Autodesk Inventor part; units mm, degrees
(part 2 of 2)
sketch "Sketch3" plane through (-0.0003, -144.9621, -142.4319) normal (0, 0, -1) x (-1, 0, 0)
  line L0 (-10.1604, 66.049) -> (-10.1604, 136.1421) construction
  line L1 (-10.1604, 136.1421) -> (-1.0068, 136.1421) construction
  line L2 (-1.0068, 136.1421) -> (-1.0068, 66.049) construction
  line L3 (-1.0068, 66.049) -> (-10.1604, 66.049) construction
  spline S0 degree 2 poles (-7.5802, 71.9161) (-7.0615, 71.9161) (-6.128, 71.5465) (-5.8038, 71.2159) knots 0 0 0 1 2 2 2
  spline S1 degree 2 poles (-5.8038, 71.2159) (-5.3954, 70.801) (-4.974, 69.6794) (-4.974, 68.8237) knots 0 0 0 1 2 2 2
  line L4 (-4.974, 68.8237) -> (-4.974, 67.9225)
  line L5 (-4.974, 67.9225) -> (-1.9918, 67.9225)
  line L6 (-1.9918, 67.9225) -> (-1.9918, 66.8593)
  line L7 (-1.9918, 66.8593) -> (-9.9918, 66.8593)
  line L8 (-9.9918, 66.8593) -> (-9.9918, 68.8691)
  spline S2 degree 2 poles (-9.9918, 68.8691) (-9.9918, 69.5822) (-9.7585, 70.5806) (-9.4927, 70.9631) knots 0 0 0 1 2 2 2
  spline S3 degree 2 poles (-9.4927, 70.9631) (-9.188, 71.4104) (-8.2479, 71.9161) (-7.5802, 71.9161) knots 0 0 0 1 2 2 2
  spline S4 degree 2 poles (-7.5478, 70.8075) (-7.9627, 70.8075) (-8.5721, 70.5222) (-8.7666, 70.2305) knots 0 0 0 1 2 2 2
  spline S5 degree 2 poles (-8.7666, 70.2305) (-8.9351, 69.9777) (-9.0713, 69.3034) (-9.0713, 68.8042) knots 0 0 0 1 2 2 2
  line L9 (-9.0713, 68.8042) -> (-9.0713, 67.9225)
  line L10 (-9.0713, 67.9225) -> (-5.8816, 67.9225)
  line L11 (-5.8816, 67.9225) -> (-5.8816, 68.6486)
  spline S6 degree 2 poles (-5.8816, 68.6486) (-5.8816, 69.2969) (-6.0891, 70.0943) (-6.3614, 70.3537) knots 0 0 0 1 2 2 2
  spline S7 degree 2 poles (-6.3614, 70.3537) (-6.6012, 70.5935) (-7.1653, 70.8075) (-7.5478, 70.8075) knots 0 0 0 1 2 2 2
  line L12 (-1.9918, 79.1187) -> (-1.9918, 77.7378)
  line L13 (-1.9918, 77.7378) -> (-5.175, 75.2094)
  line L14 (-5.175, 75.2094) -> (-5.175, 73.9906)
  line L15 (-5.175, 73.9906) -> (-1.9918, 73.9906)
  line L16 (-1.9918, 73.9906) -> (-1.9918, 72.9274)
  line L17 (-1.9918, 72.9274) -> (-9.9918, 72.9274)
  line L18 (-9.9918, 72.9274) -> (-9.9918, 74.989)
  spline S8 degree 2 poles (-9.9918, 74.989) (-9.9918, 75.6762) (-9.8427, 76.6033) (-9.5705, 77.0247) knots 0 0 0 1 2 2 2
  spline S9 degree 2 poles (-9.5705, 77.0247) (-9.2982, 77.446) (-8.4489, 77.9323) (-7.82, 77.9323) knots 0 0 0 1 2 2 2
  spline S10 degree 2 poles (-7.82, 77.9323) (-6.9448, 77.9323) (-5.7585, 77.0376) (-5.4732, 76.2726) knots 0 0 0 1 2 2 2
  line L19 (-5.4732, 76.2726) -> (-1.9918, 79.1187)
  spline S11 degree 2 poles (-7.7358, 76.8237) (-8.0858, 76.8237) (-8.6239, 76.5773) (-8.799, 76.318) knots 0 0 0 1 2 2 2
  spline S12 degree 2 poles (-8.799, 76.318) (-8.9481, 76.0911) (-9.0713, 75.4882) (-9.0713, 75.0473) knots 0 0 0 1 2 2 2
  line L20 (-9.0713, 75.0473) -> (-9.0713, 73.9906)
  line L21 (-9.0713, 73.9906) -> (-6.0632, 73.9906)
  line L22 (-6.0632, 73.9906) -> (-6.0632, 74.9242)
  spline S13 degree 2 poles (-6.0632, 74.9242) (-6.0632, 75.3845) (-6.2252, 76.117) (-6.4781, 76.3699) knots 0 0 0 1 2 2 2
  spline S14 degree 2 poles (-6.4781, 76.3699) (-6.6985, 76.6033) (-7.3209, 76.8237) (-7.7358, 76.8237) knots 0 0 0 1 2 2 2
  spline S15 degree 2 poles (-9.0777, 85.4136) (-8.5461, 85.8674) (-6.9902, 86.3731) (-5.9918, 86.3731) knots 0 0 0 1 2 2 2
  spline S16 degree 2 poles (-5.9918, 86.3731) (-5.0194, 86.3731) (-3.444, 85.8804) (-2.9124, 85.4136) knots 0 0 0 1 2 2 2
  spline S17 degree 2 poles (-2.9124, 85.4136) (-2.3549, 84.9209) (-1.8233, 83.6178) (-1.8233, 82.8334) knots 0 0 0 1 2 2 2
  spline S18 degree 2 poles (-1.8233, 82.8334) (-1.8233, 82.023) (-2.3743, 80.7264) (-2.9124, 80.2532) knots 0 0 0 1 2 2 2
  spline S19 degree 2 poles (-2.9124, 80.2532) (-3.444, 79.7929) (-5.0064, 79.3002) (-5.9918, 79.3002) knots 0 0 0 1 2 2 2
  spline S20 degree 2 poles (-5.9918, 79.3002) (-6.9967, 79.3002) (-8.5267, 79.7994) (-9.0777, 80.2597) knots 0 0 0 1 2 2 2
  spline S21 degree 2 poles (-9.0777, 80.2597) (-9.6094, 80.7264) (-10.1604, 82.0295) (-10.1604, 82.8334) knots 0 0 0 1 2 2 2
  spline S22 degree 2 poles (-10.1604, 82.8334) (-10.1604, 83.6503) (-9.5899, 84.9598) (-9.0777, 85.4136) knots 0 0 0 1 2 2 2
  spline S23 degree 2 poles (-5.9918, 85.2645) (-6.7828, 85.2645) (-8.0081, 84.9209) (-8.41, 84.6097) knots 0 0 0 1 2 2 2
  spline S24 degree 2 poles (-8.41, 84.6097) (-8.8249, 84.2921) (-9.2398, 83.3974) (-9.2398, 82.8399) knots 0 0 0 1 2 2 2
  spline S25 degree 2 poles (-9.2398, 82.8399) (-9.2398, 82.2629) (-8.8379, 81.3942) (-8.41, 81.0636) knots 0 0 0 1 2 2 2
  spline S26 degree 2 poles (-8.41, 81.0636) (-8.0016, 80.7459) (-6.7698, 80.4088) (-5.9918, 80.4088) knots 0 0 0 1 2 2 2
  spline S27 degree 2 poles (-5.9918, 80.4088) (-4.4165, 80.4088) (-2.7439, 81.7313) (-2.7439, 82.8399) knots 0 0 0 1 2 2 2
  spline S28 degree 2 poles (-2.7439, 82.8399) (-2.7439, 83.9485) (-4.4165, 85.2645) (-5.9918, 85.2645) knots 0 0 0 1 2 2 2
  line L23 (-1.9918, 89.4071) -> (-9.0453, 89.4071)
  line L24 (-9.0453, 89.4071) -> (-9.0453, 86.7232)
  line L25 (-9.0453, 86.7232) -> (-9.9918, 86.7232)
  line L26 (-9.9918, 86.7232) -> (-9.9918, 93.1543)
  line L27 (-9.9918, 93.1543) -> (-9.0453, 93.1543)
  line L28 (-9.0453, 93.1543) -> (-9.0453, 90.4704)
  line L29 (-9.0453, 90.4704) -> (-1.9918, 90.4704)
  line L30 (-1.9918, 90.4704) -> (-1.9918, 89.4071)
  spline S29 degree 2 poles (-9.0777, 99.6243) (-8.5461, 100.0781) (-6.9902, 100.5838) (-5.9918, 100.5838) knots 0 0 0 1 2 2 2
  spline S30 degree 2 poles (-5.9918, 100.5838) (-5.0194, 100.5838) (-3.444, 100.0911) (-2.9124, 99.6243) knots 0 0 0 1 2 2 2
  spline S31 degree 2 poles (-2.9124, 99.6243) (-2.3549, 99.1316) (-1.8233, 97.8285) (-1.8233, 97.0441) knots 0 0 0 1 2 2 2
  spline S32 degree 2 poles (-1.8233, 97.0441) (-1.8233, 96.2337) (-2.3743, 94.9371) (-2.9124, 94.4639) knots 0 0 0 1 2 2 2
  spline S33 degree 2 poles (-2.9124, 94.4639) (-3.444, 94.0036) (-5.0064, 93.5109) (-5.9918, 93.5109) knots 0 0 0 1 2 2 2
  spline S34 degree 2 poles (-5.9918, 93.5109) (-6.9967, 93.5109) (-8.5267, 94.0101) (-9.0777, 94.4704) knots 0 0 0 1 2 2 2
  spline S35 degree 2 poles (-9.0777, 94.4704) (-9.6094, 94.9371) (-10.1604, 96.2402) (-10.1604, 97.0441) knots 0 0 0 1 2 2 2
  spline S36 degree 2 poles (-10.1604, 97.0441) (-10.1604, 97.861) (-9.5899, 99.1705) (-9.0777, 99.6243) knots 0 0 0 1 2 2 2
  spline S37 degree 2 poles (-5.9918, 99.4752) (-6.7828, 99.4752) (-8.0081, 99.1316) (-8.41, 98.8204) knots 0 0 0 1 2 2 2
  spline S38 degree 2 poles (-8.41, 98.8204) (-8.8249, 98.5028) (-9.2398, 97.6081) (-9.2398, 97.0506) knots 0 0 0 1 2 2 2
  spline S39 degree 2 poles (-9.2398, 97.0506) (-9.2398, 96.4736) (-8.8379, 95.6049) (-8.41, 95.2742) knots 0 0 0 1 2 2 2
  spline S40 degree 2 poles (-8.41, 95.2742) (-8.0016, 94.9566) (-6.7698, 94.6195) (-5.9918, 94.6195) knots 0 0 0 1 2 2 2
  spline S41 degree 2 poles (-5.9918, 94.6195) (-4.4165, 94.6195) (-2.7439, 95.942) (-2.7439, 97.0506) knots 0 0 0 1 2 2 2
  spline S42 degree 2 poles (-2.7439, 97.0506) (-2.7439, 98.1592) (-4.4165, 99.4752) (-5.9918, 99.4752) knots 0 0 0 1 2 2 2
  line L31 (-1.9918, 103.6178) -> (-9.0453, 103.6178)
  line L32 (-9.0453, 103.6178) -> (-9.0453, 100.9339)
  line L33 (-9.0453, 100.9339) -> (-9.9918, 100.9339)
  line L34 (-9.9918, 100.9339) -> (-9.9918, 107.365)
  line L35 (-9.9918, 107.365) -> (-9.0453, 107.365)
  line L36 (-9.0453, 107.365) -> (-9.0453, 104.6811)
  line L37 (-9.0453, 104.6811) -> (-1.9918, 104.6811)
  line L38 (-1.9918, 104.6811) -> (-1.9918, 103.6178)
  line L39 (-9.9918, 113.7767) -> (-5.5316, 111.0733)
  line L40 (-5.5316, 111.0733) -> (-1.9918, 111.0733)
  line L41 (-1.9918, 111.0733) -> (-1.9918, 110.0101)
  line L42 (-1.9918, 110.0101) -> (-5.4213, 110.0101)
  line L43 (-5.4213, 110.0101) -> (-9.9918, 107.3067)
  line L44 (-9.9918, 107.3067) -> (-9.9918, 108.4866)
  line L45 (-9.9918, 108.4866) -> (-6.4716, 110.5482)
  line L46 (-6.4716, 110.5482) -> (-9.9918, 112.6486)
  line L47 (-9.9918, 112.6486) -> (-9.9918, 113.7767)
  spline S43 degree 2 poles (-7.5802, 119.5725) (-7.0615, 119.5725) (-6.128, 119.2029) (-5.8038, 118.8723) knots 0 0 0 1 2 2 2
  spline S44 degree 2 poles (-5.8038, 118.8723) (-5.3954, 118.4574) (-4.974, 117.3358) (-4.974, 116.4801) knots 0 0 0 1 2 2 2
  line L48 (-4.974, 116.4801) -> (-4.974, 115.5789)
  line L49 (-4.974, 115.5789) -> (-1.9918, 115.5789)
  line L50 (-1.9918, 115.5789) -> (-1.9918, 114.5157)
  line L51 (-1.9918, 114.5157) -> (-9.9918, 114.5157)
  line L52 (-9.9918, 114.5157) -> (-9.9918, 116.5255)
  spline S45 degree 2 poles (-9.9918, 116.5255) (-9.9918, 117.2386) (-9.7585, 118.237) (-9.4927, 118.6195) knots 0 0 0 1 2 2 2
  spline S46 degree 2 poles (-9.4927, 118.6195) (-9.188, 119.0668) (-8.2479, 119.5725) (-7.5802, 119.5725) knots 0 0 0 1 2 2 2
  spline S47 degree 2 poles (-7.5478, 118.4639) (-7.9627, 118.4639) (-8.5721, 118.1786) (-8.7666, 117.8869) knots 0 0 0 1 2 2 2
  spline S48 degree 2 poles (-8.7666, 117.8869) (-8.9351, 117.6341) (-9.0713, 116.9598) (-9.0713, 116.4606) knots 0 0 0 1 2 2 2
  line L53 (-9.0713, 116.4606) -> (-9.0713, 115.5789)
  line L54 (-9.0713, 115.5789) -> (-5.8816, 115.5789)
  line L55 (-5.8816, 115.5789) -> (-5.8816, 116.305)
  spline S49 degree 2 poles (-5.8816, 116.305) (-5.8816, 116.9533) (-6.0891, 117.7507) (-6.3614, 118.0101) knots 0 0 0 1 2 2 2
  spline S50 degree 2 poles (-6.3614, 118.0101) (-6.6012, 118.2499) (-7.1653, 118.4639) (-7.5478, 118.4639) knots 0 0 0 1 2 2 2
  line L56 (-1.9918, 120.5838) -> (-9.9918, 120.5838)
  line L57 (-9.9918, 120.5838) -> (-9.9918, 125.5887)
  line L58 (-9.9918, 125.5887) -> (-9.0453, 125.5887)
  line L59 (-9.0453, 125.5887) -> (-9.0453, 121.647)
  line L60 (-9.0453, 121.647) -> (-6.8541, 121.647)
  line L61 (-6.8541, 121.647) -> (-6.8541, 125.3229)
  line L62 (-6.8541, 125.3229) -> (-5.9076, 125.3229)
  line L63 (-5.9076, 125.3229) -> (-5.9076, 121.647)
  line L64 (-5.9076, 121.647) -> (-2.9384, 121.647)
  line L65 (-2.9384, 121.647) -> (-2.9384, 125.5887)
  line L66 (-2.9384, 125.5887) -> (-1.9918, 125.5887)
  line L67 (-1.9918, 125.5887) -> (-1.9918, 120.5838)
  line L68 (-1.9918, 134.4963) -> (-1.9918, 130.5935)
  line L69 (-1.9918, 130.5935) -> (-2.8087, 130.5935)
  line L70 (-2.8087, 130.5935) -> (-2.8087, 132.0457)
  line L71 (-2.8087, 132.0457) -> (-8.1701, 132.0457)
  line L72 (-8.1701, 132.0457) -> (-8.1701, 130.5935)
  line L73 (-8.1701, 130.5935) -> (-8.9027, 130.5935)
  spline S51 degree 2 poles (-8.9027, 130.5935) (-8.9027, 131.4169) (-9.3695, 132.1948) (-10.0178, 132.2467) knots 0 0 0 1 2 2 2
  line L74 (-10.0178, 132.2467) -> (-10.0178, 133.0765)
  line L75 (-10.0178, 133.0765) -> (-2.8087, 133.0765)
  line L76 (-2.8087, 133.0765) -> (-2.8087, 134.4963)
  line L77 (-2.8087, 134.4963) -> (-1.9918, 134.4963)
  point P0 (-0.0003, 144.9621)
  constraints: 2 other
extrude "Extrusion3" add sketch "Sketch3" against normal blind 2
body "Solid1"
